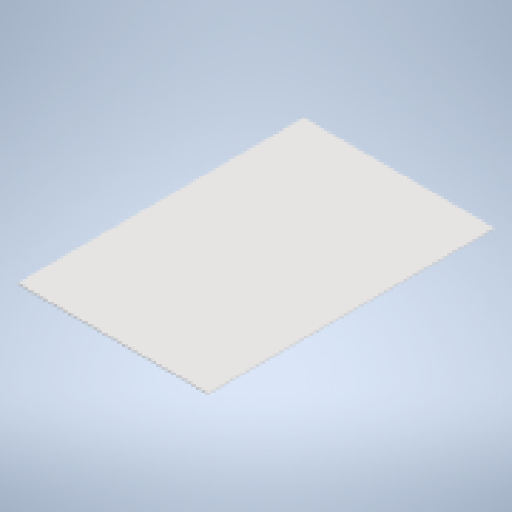
# Autodesk Inventor part: floor
Saved by Autodesk Inventor 2023.2 (Build 272271030, 271C)
## iProperties
Created: 2023-06-19
Part Number: floor
Material: Generic
Document SubType Name: Modeling
Designer: kao91
Density: 1 g/cm^3
Appearance: Default
Author: kao91
Autodesk Inventor part; units mm, degrees
ref_plane "YZ Plane" through (0, 0, 0) normal (1, 0, 0) x (0, 1, 0)
ref_plane "XZ Plane" through (0, 0, 0) normal (0, 1, 0) x (-1, 0, 0)
ref_plane "XY Plane" through (0, 0, 0) normal (0, 0, 1) x (1, 0, 0)
sketch "Sketch1" plane through (0, 0, 0) normal (0, 1, 0) x (-1, 0, 0)
  line L0 (92.6587, 169.6429) -> (-107.3413, 169.6429)
  line L1 (-107.3413, 169.6429) -> (-107.3413, -130.3571)
  line L2 (-107.3413, -130.3571) -> (92.6587, -130.3571)
  line L3 (92.6587, -130.3571) -> (92.6587, 169.6429)
  point P0 (0, 0)
  dimension "d0" = 300
  dimension "d1" = 200
  constraints: 8 end point, 2 parallel, 1 horizontal, 1 perpendicular
  measures "d0" distance of L2.end L0.start
  measures "d1" distance of L0.start L0.end
extrude "Extrusion1" add sketch "Sketch1" along normal blind 1
body "Solid1"
